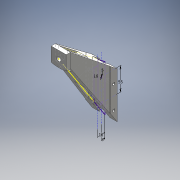
# Autodesk Inventor part: PRING_vertical_bar
Saved by Autodesk Inventor 2018 (Build 220112000, 112)
## iProperties
Created: 2026-06-13
Part Number: PRING_vertical_bar
Material: Generic
Document SubType Name: Modeling
Designer: neo
Density: 1 g/cm^3
Appearance: Default
Mass: 236.239 g
Surface Area: 521.557 cm^2
Volume: 236.239 cm^3
Author: neo
Autodesk Inventor part; units mm, degrees
ref_plane "YZ Plane" through (0, 0, 0) normal (1, 0, 0) x (0, 1, 0)
sketch "Sketch1" plane through (0, 0, 0) normal (0, 1, 0) x (-1, 0, 0)
  line L0 (18, 18) -> (-18, 18)
  line L1 (-18, 18) -> (-18, -18)
  line L2 (-1.0844, -18) -> (0, -18)
  line L3 (18, -18) -> (18, 18)
  line L4 (0, 31.7221) -> (0, -30.6703)
  line L5 (20.2298, 0) -> (-39.3416, 0)
  line L6 (18, 62) -> (-19.0844, 62) construction
  arc A0 (0, -18) -> (18, -15.8234) centre (-0.5422, 62) ccw
  arc A1 (-18, -16.0738) -> (-1.0844, -18) centre (-0.5422, 62) ccw
  circle A2 centre (0, 0) radius 5.1
  dimension "d0" = 36
  dimension "d1" = 36
  dimension "d2" = 80
  dimension "d6" = 10.2
  constraints: 14 end point, 4 point on circle, 3 centre point, 3 horizontal, 3 point on line, 2 parallel, 1 coincident, 1 midpoint, 1 perpendicular, 1 vertical, 2 other
  measures "d0" distance of L3.start L1.end
  measures "d1" distance of L3.start L0.start
  measures "d2" distance between parallel lines of L6 L2
  measures "d6" diameter of A2
extrude "Extrusion1" add sketch "Sketch1" along normal blind 10
extrude "Extrusion2" cut sketch "Sketch1" along normal through all contours A2 L5 L4 | L4 L5 A2 | A2 L4 L5 | L4 A2 L5
sketch "Sketch2" plane through (0, 10, 0) normal (0, 1, 0) x (1, 0, 0)
  circle A0 centre (0, 0) radius 5.1 construction
  line L0 (-18, -18) -> (18, -18) construction
  line L1 (18, -18) -> (18, 16.0738) construction
  arc A1 (18, 16.0738) -> (1.0844, 18) centre (0.5422, -62) ccw construction
  line L2 (1.0844, 18) -> (0, 18) construction
  arc A2 (0, 18) -> (-18, 15.8234) centre (0.5422, -62) ccw construction
  line L3 (-18, 15.8234) -> (-18, -18) construction
  line L4 (18, -18) -> (10, -18)
  line L5 (10, -18) -> (10, 15.8234)
  line L6 (10, 15.8234) -> (18, 15.8234)
  line L7 (18, 15.8234) -> (18, -18)
  dimension "d9" = 8
  constraints: 8 end point, 2 parallel, 1 horizontal, 1 perpendicular
  measures "d9" distance between parallel lines of L1 L5
ref_plane "height_panel" through (0, 110, 0) normal (0, 1, 0) x (1, 0, 0)
sketch "Sketch3" plane through (0, 110, 0) normal (0, 1, 0) x (1, 0, 0)
  line L0 (15, 60) -> (30, 60)
  line L1 (30, 60) -> (30, 170)
  line L2 (30, 170) -> (15, 170)
  line L3 (15, 170) -> (15, 60)
  line L4 (0, -34.344) -> (0, 41.1374) construction
  circle A0 centre (0, 0) radius 5.1 construction
  line L5 (0, 0) -> (37.0806, 0) construction
  line L6 (0, 0) -> (-113.2425, 196.1417) construction
  line L7 (0, 0) -> (113.2425, 196.1417) construction
  dimension "d15" = 15
  dimension "d16" = 110
  dimension "d17" = 30
  dimension "d18" = 0
  dimension "d20" = 60
  dimension "d23" = 60
  constraints: 16 end point, 2 coincident, 2 horizontal, 2 parallel, 1 perpendicular, 1 vertical
  measures "d15" distance of L0.start L0.end
  measures "d16" distance of L2.end L0.start
  measures "d17" distance between parallel lines of L4 L1
  measures "d18" distance from line of L4 L5.start
  measures "d20" distance between parallel lines of L5 L0
  measures "d23" angle of L7 L6
loft "support_panel" add profiles "Sketch2", "Sketch3"
ref_plane "Work Plane2" through (0, 0, -15.8234) normal (-1, 0, 0) x (0, 0, 1)
mirror "Mirror1" about plane through (0, 0, -15.8234) normal (-1, 0, 0) of "support_panel"
sketch "Sketch4" plane through (0, 0, -15.8234) normal (-1, 0, 0) x (0, 0, 1)
  line L0 (0, 10) -> (33.8234, 10) construction
  line L1 (33.8234, 10) -> (-44.1766, 110) construction
  line L2 (-154.1766, 110) -> (-44.1766, 110) construction
  line L3 (0, 10) -> (-154.1766, 110) construction
  line L4 (0, 10) -> (-154.1766, 110) projected
  line L5 (-61.6706, 50) -> (-42.7634, 108.1882)
  line L6 (33.8234, 10) -> (-44.1766, 110) projected
  line L7 (-3.2973, 57.5907) -> (-15.4177, 20)
  line L8 (-42.7634, 108.1882) -> (-3.2973, 57.5907)
  line L9 (-61.6706, 50) -> (-15.4177, 20)
  point P0 (15.8234, 0)
  dimension "d24" = 60
  dimension "d25" = 90
  constraints: 8 end point, 4 point on line, 2 collinear
  measures "d24" distance from line of L2 L5.start
  measures "d25" distance from line of L7.end L2
extrude "Extrusion3" add sketch "Sketch4" along normal mid plane 38
sketch "Sketch5" plane through (0, 0, -15.8234) normal (-1, 0, 0) x (0, 0, 1)
  line L0 (-20.1302, 94) -> (-176.0391, 94) construction
  line L1 (-154.1766, 110) -> (-44.1766, 110) construction
  line L2 (-18.8309, 102) -> (-169.7053, 102) construction
  line L3 (33.8234, 10) -> (-44.1766, 110) construction
  line L4 (-44.1766, 110) -> (-44.1766, 74.3483) construction
  line L5 (-71.6766, 137.3856) -> (-71.6766, 103.9302) construction
  line L6 (-126.6766, 137.3856) -> (-126.6766, 97.2716) construction
  line L7 (-44.1766, 110) -> (-154.1766, 110) construction
  line L8 (-99.1766, 110) -> (-99.1766, 73.2356) construction
  circle A0 centre (-71.6766, 102) radius 2.5 construction
  line L9 (-69.1766, 104.5) -> (-74.1766, 104.5)
  line L10 (-74.1766, 104.5) -> (-74.1766, 99.5)
  line L11 (-74.1766, 99.5) -> (-69.1766, 99.5)
  line L12 (-69.1766, 99.5) -> (-69.1766, 104.5)
  circle A1 centre (-126.6766, 102) radius 2.5 construction
  line L13 (-129.1766, 104.5) -> (-124.1766, 104.5)
  line L14 (-124.1766, 104.5) -> (-124.1766, 99.5)
  line L15 (-124.1766, 99.5) -> (-129.1766, 99.5)
  line L16 (-129.1766, 99.5) -> (-129.1766, 104.5)
  line L17 (-44.1766, 110) -> (-31.6966, 94)
  line L18 (0, 10) -> (-154.1766, 110) projected
  line L19 (-129.5083, 94) -> (-154.1766, 110)
  line L20 (-154.1766, 110) -> (-44.1766, 110)
  line L21 (-31.6966, 94) -> (-129.5083, 94)
  line L22 (-44.1766, 94) -> (-129.5083, 94)
  line L23 (-44.1766, 94) -> (-44.1766, 84)
  line L24 (-44.1766, 84) -> (-114.0907, 84)
  line L25 (-114.0907, 84) -> (-129.5083, 94)
  line L26 (-44.1766, 94) -> (-129.5083, 94)
  point P0 (15.8234, 0)
  dimension "d28" = 16
  dimension "d29" = 8
  dimension "d30" = 55
  dimension "d31" = 5
  dimension "d40" = 10
  constraints: 46 end point, 11 point on line, 6 collinear, 5 symmetric about line, 4 vertical, 3 horizontal, 3 perpendicular, 3 tangent, 2 centre point, 2 parallel, 1 midpoint, 2 other
  measures "d28" distance between parallel lines of L0 L1
  measures "d29" distance between parallel lines of L2 L1
  measures "d30" distance between parallel lines of L6 L5
  measures "d31" diameter of A0
  measures "d40" distance between parallel lines of L0 L24
extrude "Extrusion5" add sketch "Sketch5" along normal mid plane 60 contours L17 L21 L18 L20
extrude "installation_rack" cut sketch "Sketch5" along normal mid plane 25 contours L17 L21 L18 L20
extrude "Extrusion7" cut sketch "Sketch5" along normal through all both and the other way through all contours L12 L11 L10 L9 | L13 L14 L15 L16
extrude "Extrusion8" add sketch "Sketch5" along normal mid plane 30 contours L23 L24 L18 L21
body "Solid1"
